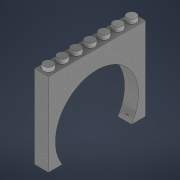
# Autodesk Inventor part: 110033226_ipt_22_塔樓門口
Saved by Autodesk Inventor 2022 (Build 260153000, 153)
## iProperties
Created: 2022-06-23
Part Number: 110033226_ipt_22_塔樓門口
Material: 一般
Document SubType Name: Modeling
Designer: User
Density: 1 g/cm^3
Appearance: 預設
Author: User
Autodesk Inventor part; units mm, degrees
ref_plane "YZ Plane" through (0, 0, 0) normal (1, 0, 0) x (0, 1, 0)
ref_plane "XZ Plane" through (0, 0, 0) normal (0, 1, 0) x (-1, 0, 0)
ref_plane "XY Plane" through (0, 0, 0) normal (0, 0, 1) x (1, 0, 0)
sketch "草圖1" plane through (0, 0, 0) normal (0, 1, 0) x (-1, 0, 0)
  line L0 (5, 0) -> (0, 0)
  line L1 (0, 0) -> (0, -35)
  line L2 (0, -35) -> (5, -35)
  line L3 (5, -35) -> (5, 0)
  circle A0 centre (2.5, -2.5) radius 1.7
  circle A1 centre (2.5, -7.5) radius 1.7
  circle A2 centre (2.5, -12.5) radius 1.7
  circle A3 centre (2.5, -17.5) radius 1.7
  circle A4 centre (2.5, -22.5) radius 1.7
  circle A5 centre (2.5, -27.5) radius 1.7
  circle A6 centre (2.5, -32.5) radius 1.7
  line L4 (5, -5) -> (0, -5)
  line L5 (5, -30) -> (0, -30)
  dimension "d0" = 5
  dimension "d1" = 35
  dimension "d2" = 3.4
  dimension "d3" = 2.5
  dimension "d4" = 2.5
  dimension "d7" = 5
  dimension "d12" = 5
  dimension "d13" = 5
  constraints: 12 end point, 7 centre point, 4 point on line, 3 perpendicular, 2 parallel, 1 coincident, 1 horizontal, 1 vertical, 12 other
  measures "d0" distance of L2.end L1.end
  measures "d1" distance of L1.end L0.end
  measures "d2" diameter of A0
  measures "d3" distance from line of L1 A0.centre
  measures "d4" distance from line of L0 A0.centre
  measures "d7" distance of A0.centre A1.centre
  measures "d12" distance between parallel lines of L2 L5
  measures "d13" distance between parallel lines of L0 L4
sketch "草圖2" plane through (0, 0, 0) normal (1, 0, 0) x (0, 1, 0)
  line L0 (0, 0) -> (0, -35) projected
  line L1 (0, 0) -> (30, 0)
  line L2 (30, 0) -> (30, -35)
  line L3 (30, -35) -> (0, -35)
  arc A0 (0, -30) -> (0, -5) centre (8.2916, -17.5) ccw
  point P0 (0, -5)
  dimension "d15" = 30
  dimension "d25" = 15
  constraints: 6 end point, 2 point on circle, 1 centre point, 1 horizontal, 1 perpendicular, 1 vertical, 1 other
  measures "d15" distance of L1.start L1.end
  measures "d25" radius of A0
extrude "擠出1" add sketch "草圖2" against normal blind 5 contours L1 L2 L3 L0 A0
extrude "擠出2" cut sketch "草圖1" along normal blind 1.5 contours A0 | A6
sketch "草圖3" plane through (0, 30, 0) normal (0, 1, 0) x (1, 0, 0)
  arc A0 (-2.9974, 4.1256) -> (-2.0026, 4.1256) centre (-2.5, 2.5) ccw projected
  circle A1 centre (-2.5, 2.5) radius 1.7
  point P0 (0, 0)
  point P1 (-2.9974, 4.1256)
  constraints: 1 centre point, 1 coincident, 1 concentric
extrude "擠出4" add sketch "草圖3" along normal blind 1.5
pattern_linear "矩形陣列2" count 7 spacing 5 along (0, 0, -1) of "擠出4"
